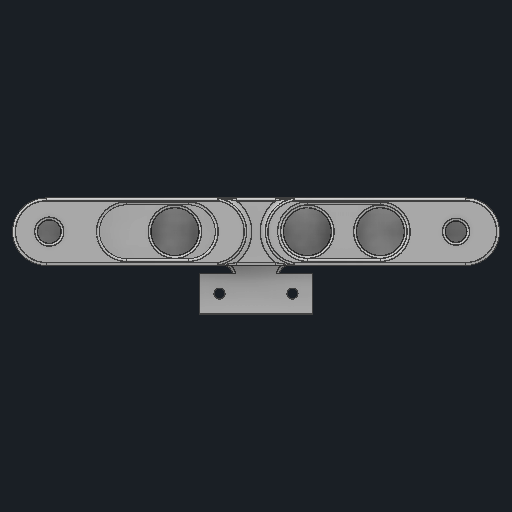
# Autodesk Inventor part: PrimeSenseCarmine1.09
Saved by Autodesk Inventor 2025.2 (Build 292293000, 293)
## iProperties
Created: 2024-11-08
Part Number: PrimeSenseCarmine1.09
Material: Generic
Document SubType Name: Modeling
Designer: valer
Density: 1 g/cm^3
Appearance: Default
Author: valer
Autodesk Inventor part; units mm, degrees
ref_plane "YZ Plane" through (0, 0, 0) normal (1, 0, 0) x (0, 1, 0)
ref_plane "XZ Plane" through (0, 0, 0) normal (0, 1, 0) x (-1, 0, 0)
ref_plane "XY Plane" through (0, 0, 0) normal (0, 0, 1) x (1, 0, 0)
sketch "Sensor" plane through (0, 0, 0) normal (0, 0, 1) x (1, 0, 0)
  circle A0 centre (19, 0) radius 8.875
  circle A1 centre (46, 0) radius 8.875
  circle A2 centre (-30, 0) radius 8.875
  circle A3 centre (-76.5, 0) radius 4.375
  line L0 (-90, 12.415) -> (90, 12.415)
  line L1 (90, 12.415) -> (90, -12.415)
  line L2 (90, -12.415) -> (-90, -12.415)
  line L3 (-90, -12.415) -> (-90, 12.415)
  line L4 (-90, 0) -> (90, 0) construction
  arc A4 (-77.585, 12.415) -> (-77.585, -12.415) centre (-77.585, 0) ccw
  arc A5 (77.585, -12.415) -> (77.585, 12.415) centre (77.585, 0) ccw
  circle A6 centre (74, 0) radius 4
  point P0 (0, 0)
  point P1 (0, 0)
  dimension "d0" = 17.75
  dimension "d1" = 180
  dimension "d2" = 24.83
  dimension "d3" = 8.75
  dimension "d4" = 46
  dimension "d5" = 27
  dimension "d6" = 30
  dimension "d7" = 13.5
  dimension "d8" = 16
  dimension "d9" = 8
  constraints: 8 end point, 7 centre point, 4 point on circle, 4 point on line, 4 tangent, 2 equal radius, 2 midpoint, 2 parallel, 1 coincident, 1 horizontal, 1 perpendicular, 11 other
  measures "d0" diameter of A0
  measures "d1" distance of L0.start L0.end
  measures "d2" distance of L2.end L0.start
  measures "d3" diameter of A3
  measures "d4" distance of point (0, 0) A1.centre
  measures "d5" distance of A1.centre A0.centre
  measures "d6" distance of point (0, 0) A2.centre
  measures "d7" distance from line of A3.centre L3
  measures "d8" distance from line of L1 A6.centre
  measures "d9" diameter of A6
extrude "SensorFeature" add sketch "Sensor" along normal blind 35.94 contours L0 A5 L2 A4
sketch "Sketch2" plane through (0, 0, 0) normal (0, 0, -1) x (-1, 0, 0)
  line L0 (-77.585, 12.415) -> (77.585, 12.415) projected
  arc A0 (-77.585, 12.415) -> (-77.585, -12.415) centre (-77.585, 0) ccw projected
  line L1 (77.585, -12.415) -> (-77.585, -12.415) projected
  arc A1 (77.585, -12.415) -> (77.585, 12.415) centre (77.585, 0) ccw projected
  point P0 (0, 0)
extrude "Extrusion2" add sketch "Sketch2" against normal blind 10
sketch "Sketch3" plane through (-77.585, -12.415, 0) normal (0, -1, 0) x (1, 0, 0)
  line L0 (69.17, 25.545) -> (86, 25.545)
  line L1 (86, 25.545) -> (86, 10.395)
  line L2 (86, 10.395) -> (69.17, 10.395)
  line L3 (69.17, 10.395) -> (69.17, 25.545)
  line L4 (0, 35.94) -> (155.17, 35.94) projected
  line L5 (77.585, 35.94) -> (77.585, 0) construction
  line L6 (0, 0) -> (155.17, 0) projected
  point P0 (77.585, 25.545)
  dimension "d14" = 16.83
  dimension "d15" = 15.15
  dimension "d16" = 10.395
  dimension "d17" = 10.395
  constraints: 10 end point, 2 midpoint, 2 parallel, 1 horizontal, 1 perpendicular, 1 point on line, 1 vertical
  measures "d14" distance of L1.end L2.end
  measures "d15" distance between parallel lines of L2 L0
  measures "d16" distance between parallel lines of L4 L0
  measures "d17" distance between parallel lines of L6 L2
extrude "Extrusion3" add sketch "Sketch3" along normal blind 18.7
sketch "Sketch4" plane through (-8.415, -12.415, 25.545) normal (0, 0, 1) x (1, 0, 0)
  line L0 (-41.585, -22.7) -> (58.415, -22.7)
  line L1 (58.415, -22.7) -> (58.415, -18.7)
  line L2 (58.415, -18.7) -> (-41.585, -18.7)
  line L3 (-41.585, -18.7) -> (-41.585, -22.7)
  line L4 (0, -18.7) -> (16.83, -18.7) construction
  line L5 (8.415, -18.7) -> (8.415, 0) construction
  line L6 (16.83, 0) -> (0, 0) construction
  line L7 (16.83, -18.7) -> (0, -18.7) projected
  point P0 (8.415, 12.415)
  dimension "d20" = 100
  dimension "d21" = 4
  constraints: 10 end point, 4 midpoint, 2 parallel, 1 horizontal, 1 perpendicular
  measures "d20" distance of L0.start L0.end
  measures "d21" distance of L2.end L0.start
ref_plane "Work Plane1" through (-8.415, -12.415, 17.97) normal (0, 0, 1) x (1, 0, 0)
sketch "Sketch5" plane through (-8.415, -12.415, 17.97) normal (0, 0, 1) x (1, 0, 0)
  line L0 (58.415, -18.7) -> (-41.585, -18.7) projected
  line L1 (-41.585, -22.7) -> (58.415, -22.7) projected
  line L2 (-41.585, -18.7) -> (-41.585, -22.7) projected
  line L3 (58.415, -22.7) -> (58.415, -18.7) projected
  point P0 (8.415, 12.415)
extrude "Extrusion4" add sketch "Sketch5" along normal mid plane 40
sketch "Sketch6" plane through (-50, -35.115, 37.97) normal (0, -1, 0) x (1, 0, 0)
  line L0 (100, -40) -> (100, 0) projected
  line L1 (0, 0) -> (100, 0) projected
  line L2 (0, -40) -> (0, 0) projected
  line L3 (100, -40) -> (0, -40) projected
  arc A0 (20, 0) -> (20, -40) centre (20, -20) ccw
  line L4 (0, -40) -> (100, -40) projected
  line L5 (50, -40) -> (50, 0) construction
  line L6 (100, 0) -> (0, 0) projected
  arc A1 (80, -40) -> (80, 0) centre (80, -20) ccw
  point P0 (50, -37.97)
  point P1 (100, -20)
  point P2 (0, -20)
  constraints: 4 point on circle, 3 symmetric about line, 3 tangent, 2 centre point, 2 end point, 2 midpoint, 2 point on line, 1 other
extrude "Extrusion5" cut sketch "Sketch6" against normal up to surface (4 mm away) contours L3 A1 L0 | A1 L1 L0 | L3 L2 A0 | A0 L2 L1
chamfer "Chamfer1" distance 4 angle 45 4 edges at (0, 12.415, 0) (-90, 0, 0) (0, -12.415, 0) (90, 0, 0)
sketch "Sketch7" plane through (0, 0, 35.94) normal (0, 0, 1) x (1, 0, 0)
  circle A0 centre (-30, 0) radius 8.875 construction
  circle A1 centre (19, 0) radius 8.875 construction
  circle A2 centre (46, 0) radius 8.875 construction
  circle A3 centre (-25, 0) radius 10
  line L0 (-25, 0) -> (-30, 0)
  circle A4 centre (-48, 0) radius 10
  line L1 (-48, 0) -> (-30, 0) construction
  line L2 (-48, 10) -> (-25, 10)
  line L3 (-48, -10) -> (-25, -10)
  circle A5 centre (19, 0) radius 10
  circle A6 centre (46, 0) radius 10
  line L4 (19, 10) -> (46, 10)
  line L5 (19, -10) -> (46, -10)
  point P0 (0, 0)
  dimension "d29" = 20
  dimension "d30" = 5
  dimension "d31" = 18
  constraints: 12 end point, 8 point on circle, 6 tangent, 4 centre point, 3 equal radius, 2 coincident, 1 collinear, 1 horizontal, 1 parallel
  measures "d29" diameter of A3
  measures "d30" distance of L0.start L0.end
  measures "d31" distance of L1.start L0.end
extrude "Extrusion6" cut sketch "Sketch7" against normal blind 3
chamfer "Chamfer2" distance 1 angle 45 5 edges at (-80.875, 0, 35.94) (70, 0, 35.94) (37.125, 0, 32.94) (10.125, 0, 32.94) (-38.875, 0, 32.94)
chamfer "Chamfer3" distance 3 angle 45 4 edges at (0, -31.115, 37.97) (-50, -31.115, 17.97) (0, -31.115, -2.03) (50, -31.115, 17.97)
fillet "Fillet1" radius 4 4 edges at (-8.415, -31.115, 17.97) (8.415, -31.115, 17.97) (8.415, -12.415, 17.97) (-8.415, -12.415, 17.97)
fillet "Fillet2" radius 1 4 edges at (-47, -31.115, 17.97) (0, -31.115, 0.97) (47, -31.115, 17.97) (0, -31.115, 34.97)
fillet "Fillet3" radius 1 12 edges at (-9.5866, -29.9434, 25.545) (-9.5866, -13.5866, 25.545) (-8.415, -21.765, 25.545) (9.5866, -29.9434, 25.545) (9.5866, -13.5866, 25.545) (8.415, -21.765, 25.545) (-9.5866, -29.9434, 10.395) (-9.5866, -13.5866, 10.395) (-8.415, -21.765, 10.395) (9.5866, -29.9434, 10.395) (9.5866, -13.5866, 10.395) (8.415, -21.765, 10.395)
sketch "Sketch8" plane through (0, 0, 35.94) normal (0, 0, 1) x (1, 0, 0)
  circle A0 centre (16, 0) radius 12.415
  line L0 (0, 0) -> (90, 0) construction
  arc A1 (77.585, -12.415) -> (77.585, 12.415) centre (77.585, 0) ccw projected
  line L1 (77.585, 12.415) -> (-77.585, 12.415) construction
  line L2 (0, 0) -> (0, 12.415) construction
  line L3 (-77.585, 12.415) -> (77.585, 12.415) projected
  circle A2 centre (-16, 0) radius 12.415
  arc A3 (77.585, -12.415) -> (77.585, 12.415) centre (77.585, 0) ccw projected
  line L4 (16, 12.415) -> (77.585, 12.415)
  line L5 (16, -12.415) -> (77.585, -12.415)
  arc A4 (-77.585, 12.415) -> (-77.585, -12.415) centre (-77.585, 0) ccw projected
  line L6 (-77.585, 12.415) -> (-16, 12.415)
  line L7 (-77.585, -12.415) -> (-16, -12.415)
  line L8 (77.585, -12.415) -> (-77.585, -12.415) projected
  dimension "d45" = 16
  constraints: 12 end point, 5 point on circle, 5 tangent, 4 point on line, 3 horizontal, 2 centre point, 1 midpoint, 1 symmetric about line, 1 other
  measures "d45" distance of A0.centre L0.start
extrude "Extrusion7" cut sketch "Sketch8" against normal blind 2 contours A0 L8 A2 L3
fillet "Fillet4" radius 2 2 edges at (-3.585, 0, 33.94) (3.585, 0, 33.94)
fillet "Fillet5" radius 1 8 edges at (-15, 0, 35.94) (-36.5, -10, 35.94) (-58, 0, 35.94) (-36.5, 10, 35.94) (56, 0, 35.94) (32.5, -10, 35.94) (9, 0, 35.94) (32.5, 10, 35.94)
fillet "Fillet6" radius 1 4 edges at (-3.585, 0, 35.94) (-90, 0, 35.94) (-46.7925, -12.415, 35.94) (-46.7925, 12.415, 35.94)
fillet "Fillet7" radius 1 4 edges at (90, 0, 35.94) (46.7925, -12.415, 35.94) (46.7925, 12.415, 35.94) (3.585, 0, 35.94)
fillet "Fillet8" radius 1 14 edges at (-13.9642, -11.9923, 35.7565) (-11.0734, -12.415, 34.2429) (0, -12.415, 33.94) (11.0734, -12.415, 34.2429) (13.7805, -12.4017, 35.1027) (13.9642, -11.9923, 35.7565) (-13.7805, -12.4017, 35.1027) (11.0734, 12.415, 34.2429) (13.7105, 12.4073, 35.0643) (13.9642, 11.9923, 35.7565) (-10.9962, 12.415, 34.2254) (-13.7105, 12.4073, 35.0643) (-13.9642, 11.9923, 35.7565) (0, 12.415, 33.94)
split "Sculpt1" plane through (-77.585, -15.415, 4) removes the side toward (0, -1, 0)
ref_plane "Work Plane2" through (-77.585, -15.415, 4) normal (0, -1, 0) x (1, 0, 0)
sketch "Sketch9" plane through (-9.415, -12.415, 25.545) normal (0, 0, 1) x (1, 0, 0)
  line L0 (30.415, -3) -> (-11.585, -3)
  line L1 (-11.585, -3) -> (-11.585, -18)
  line L2 (-11.585, -18) -> (30.415, -18)
  line L3 (30.415, -18) -> (30.415, -3)
  line L4 (16.931, -3) -> (1.899, -3) projected
  line L5 (-11.585, -3) -> (3.415, -3) construction
  line L6 (3.415, -3) -> (3.415, -18) construction
  line L7 (3.415, -18) -> (-11.585, -18) construction
  line L8 (-11.585, -18) -> (-11.585, -3) construction
  line L9 (9.415, -3) -> (9.415, -18) construction
  line L10 (15.415, -3) -> (15.415, -18) construction
  line L11 (-11.585, -3) -> (3.415, -18) construction
  line L12 (15.415, -18) -> (30.415, -3) construction
  circle A0 centre (-4.085, -10.5) radius 2
  circle A1 centre (22.915, -10.5) radius 2
  point P0 (9.415, 12.415)
  dimension "d55" = 42
  dimension "d56" = 15
  dimension "d57" = 15
  dimension "d58" = 4
  dimension "d59" = 4
  constraints: 24 end point, 5 midpoint, 4 parallel, 2 centre point, 2 horizontal, 2 perpendicular, 2 symmetric about line, 1 collinear
  measures "d55" distance of L1.end L2.end
  measures "d56" distance of L6.end L7.end
  measures "d57" distance of L5.end L6.end
  measures "d58" diameter of A0
  measures "d59" diameter of A1
extrude "Extrusion8" add sketch "Sketch9" against normal up to surface (15.15 mm away)
equation "\"d17\" = d16"
body "Solid1"
